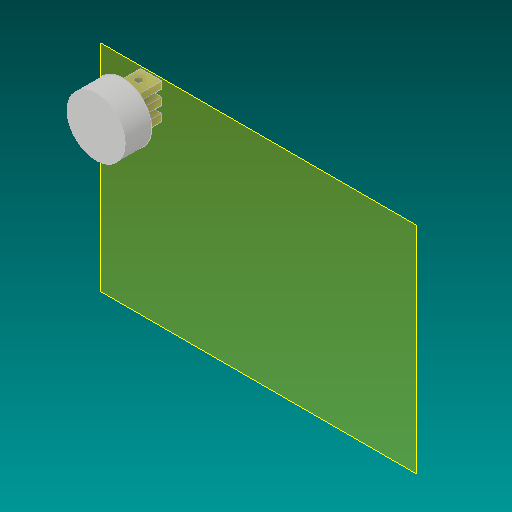
# Autodesk Inventor part: Swing_Joint
Saved by Autodesk Inventor 2019 (Build 230136000, 136)
## iProperties
Created: 2020-12-14
Part Number: Swing_Joint
Material: Generic
Document SubType Name: Modeling
Designer: Jason
Density: 1 g/cm^3
Appearance: Default
Mass: 7.44674 g
Surface Area: 30.5651 cm^2
Volume: 7.44674 cm^3
Author: Jason
Autodesk Inventor part; units mm, degrees
ref_plane "YZ Plane" through (0, 0, 0) normal (1, 0, 0) x (0, 1, 0)
ref_plane "XZ Plane" through (0, 0, 0) normal (0, 1, 0) x (-1, 0, 0)
ref_plane "XY Plane" through (0, 0, 0) normal (0, 0, 1) x (1, 0, 0)
ref_plane "Work Plane2" through (30.8055, -26.6615, 12.7) normal (0, 0, 1) x (1, 0, 0)
sketch "Sketch2" plane through (30.8055, -26.6615, 12.7) normal (0, 0, 1) x (1, 0, 0)
  circle A0 centre (-30.8055, 26.6615) radius 13
  dimension "d0" = 26
  constraints: 1 centre point, 1 coincident
  measures "d0" diameter of A0
extrude "Extrusion1" add sketch "Sketch2" along normal blind 12
sketch "Sketch5" plane through (0, 0, 12.7) normal (0, 0, -1) x (-1, 0, 0)
  line L0 (-4.7625, 7.9375) -> (4.7509, 7.9375)
  line L1 (4.7509, 7.9375) -> (4.7509, 4.7625)
  line L2 (4.7509, 4.7625) -> (-4.7625, 4.7625)
  line L3 (-4.7625, 4.7625) -> (-4.7625, 7.9375)
  line L4 (-4.7625, 1.5875) -> (4.7509, 1.5875)
  line L5 (4.7509, 1.5875) -> (4.7509, -1.5875)
  line L6 (4.7509, -1.5875) -> (-4.7625, -1.5875)
  line L7 (-4.7625, -1.5875) -> (-4.7625, 1.5875)
  line L8 (-4.7672, -4.7625) -> (4.7509, -4.7625)
  line L9 (4.7509, -4.7625) -> (4.7509, -7.9375)
  line L10 (4.7509, -7.9375) -> (-4.7672, -7.9375)
  line L11 (-4.7672, -7.9375) -> (-4.7672, -4.7625)
  point P0 (0, 0)
  constraints: 24 end point, 6 parallel, 3 horizontal, 3 perpendicular, 2 collinear
extrude "Extrusion4" add sketch "Sketch5" along normal blind 12.7
sketch "Sketch8" plane through (-4.7509, -7.9375, 12.7) normal (0, -1, 0) x (1, 0, 0)
  circle A0 centre (3.9555, -7.9375) radius 1.5875
  line L0 (9.5181, 0) -> (9.5181, -12.7) projected
  point P0 (4.7509, -12.7)
  dimension "d17" = 5.5626
  constraints: 1 centre point
  measures "d17" distance from line of A0.centre L0
extrude "Extrusion7" cut sketch "Sketch8" against normal blind 25.4
body "Solid1"
